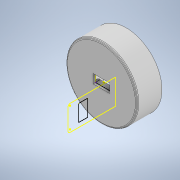
# Autodesk Inventor part: Base
Saved by Autodesk Inventor 2020 (Build 240168000, 168)
## iProperties
Created: 2020-02-27
Part Number: Base
Material: Generic
Document SubType Name: Modeling
Designer: othscs164
Density: 1 g/cm^3
Appearance: Default
Author: othscs164
Autodesk Inventor part; units mm, degrees
ref_plane "YZ Plane" through (0, 0, 0) normal (1, 0, 0) x (0, 1, 0)
ref_plane "XZ Plane" through (0, 0, 0) normal (0, 1, 0) x (-1, 0, 0)
ref_plane "XY Plane" through (0, 0, 0) normal (0, 0, 1) x (1, 0, 0)
sketch "Sketch1" plane through (0, 0, 0) normal (0, 0, 1) x (1, 0, 0)
  circle A0 centre (0, 0) radius 41.275
  circle A1 centre (0, 0) radius 47.625
  dimension "d0" = 82.55
  dimension "d1" = 6.35
  constraints: 2 centre point, 1 coincident
  measures "d0" diameter of A0
  measures "d1" radial gap between concentric circles of A0 A1
extrude "Extrusion1" add sketch "Sketch1" along normal blind 25.4
sketch "Sketch2" plane through (0, 0, 25.4) normal (0, 0, 1) x (1, 0, 0)
  circle A0 centre (0, 0) radius 47.625
  constraints: 1 centre point, 1 coincident
extrude "Extrusion2" add sketch "Sketch2" along normal blind 3.175
sketch "Sketch3" plane through (0, 0, 25.4) normal (0, 0, -1) x (-1, 0, 0)
  line L0 (11, 6) -> (-11, 6)
  line L1 (-11, 6) -> (-11, -6)
  line L2 (-11, -6) -> (11, -6)
  line L3 (11, -6) -> (11, 6)
  line L4 (11, 6) -> (-11, -6) construction
  line L5 (-11, 6) -> (11, -6) construction
  line L6 (-10.6662, 8.8412) -> (10.6662, 8.8412)
  line L7 (13.8412, 5.6662) -> (13.8412, -5.6662)
  line L8 (10.6662, -8.8412) -> (-10.6662, -8.8412)
  line L9 (-13.8412, -5.6662) -> (-13.8412, 5.6662)
  arc A0 (-10.6662, 8.8412) -> (-13.8412, 5.6662) centre (-10.6662, 5.6662) ccw
  arc A1 (-13.8412, -5.6662) -> (-10.6662, -8.8412) centre (-10.6662, -5.6662) ccw
  arc A2 (10.6662, -8.8412) -> (13.8412, -5.6662) centre (10.6662, -5.6662) ccw
  arc A3 (13.8412, 5.6662) -> (10.6662, 8.8412) centre (10.6662, 5.6662) ccw
  point P0 (0, 0)
  dimension "d6" = 22
  dimension "d7" = 12
  dimension "d8" = 3.175
  constraints: 20 end point, 8 point on circle, 8 tangent, 4 centre point, 4 parallel, 3 equal radius, 2 midpoint, 2 perpendicular, 1 horizontal, 3 other
  measures "d6" distance of L2.end L1.end
  measures "d7" distance of L1.end L0.end
  measures "d8" radius of A0
extrude "Extrusion3" add sketch "Sketch3" along normal blind 6.35
chamfer "Chamfer1" distance 1.5875 angle 45 8 edges at (0, 8.8412, 19.05) (12.9113, 7.9113, 19.05) (13.8412, 0, 19.05) (12.9113, -7.9113, 19.05) (0, -8.8412, 19.05) (-12.9113, -7.9113, 19.05) (-13.8412, 0, 19.05) (-12.9113, 7.9113, 19.05)
sketch "Sketch5" plane through (-13.8412, -5.6662, 25.4) normal (-1, 0, 0) x (0, 0, 1)
  line L0 (-0.1094, 0) -> (-8.0486, 0)
  line L1 (-8.0486, 0) -> (-8.0486, 11.3324)
  line L2 (-8.0486, 11.3324) -> (-0.1094, 11.3324)
  line L3 (-0.1094, 11.3324) -> (-0.1094, 0)
  point P0 (-25.4, 5.6662)
  constraints: 8 end point, 2 parallel, 1 horizontal, 1 perpendicular
extrude "Extrusion5" cut sketch "Sketch5" against normal blind 28.575
sketch "Sketch6" plane through (0, 0, 0) normal (0, 0, -1) x (-1, 0, 0)
  circle A0 centre (0, 0) radius 47.625 projected
  circle A1 centre (0, 0) radius 41.275 projected
extrude "Extrusion6" add sketch "Sketch6" along normal blind 4.5
chamfer "Chamfer2" distance 1.5875 angle 45 1 edges at (-47.625, 0, 28.575)
fillet "Fillet2" radius 1.5875 1 edges at (-46.0375, 0, 28.575)
fillet "Fillet3" radius 1.5875 1 edges at (-47.625, 0, 26.9875)
sketch "Sketch7" plane through (0, 0, 25.4) normal (0, 0, -1) x (-1, 0, 0)
  circle A0 centre (0, 0) radius 41.275 projected
  line L0 (-10.6662, 8.8412) -> (10.6662, 8.8412) projected
  arc A1 (13.8412, 5.6662) -> (10.6662, 8.8412) centre (10.6662, 5.6662) ccw projected
  line L1 (13.8412, 5.6662) -> (13.8412, -5.6662) projected
  arc A2 (10.6662, -8.8412) -> (13.8412, -5.6662) centre (10.6662, -5.6662) ccw projected
  line L2 (10.6662, -8.8412) -> (-10.6662, -8.8412) projected
  arc A3 (-13.8412, -5.6662) -> (-10.6662, -8.8412) centre (-10.6662, -5.6662) ccw projected
  line L3 (-13.8412, -5.6662) -> (-13.8412, 5.6662) projected
  arc A4 (-10.6662, 8.8412) -> (-13.8412, 5.6662) centre (-10.6662, 5.6662) ccw projected
  line L4 (10.6662, 7.2537) -> (10.6662, 8.8412) projected
  arc A5 (12.2537, 5.6662) -> (10.6662, 7.2537) centre (10.6662, 5.6662) ccw projected
  line L5 (13.8412, 5.6662) -> (12.2537, 5.6662) projected
  arc A6 (13.8412, 5.6662) -> (10.6662, 8.8412) centre (10.6662, 5.6662) ccw projected
  line L6 (-10.6662, 7.2537) -> (10.6662, 7.2537) projected
  line L7 (-12.2537, 5.6662) -> (-11, 5.6662) projected
  line L8 (-11, 5.6662) -> (-11, 6) projected
  line L9 (-11, 6) -> (11, 6) projected
  line L10 (11, 6) -> (11, 5.6662) projected
  line L11 (11, 5.6662) -> (12.2537, 5.6662) projected
  arc A7 (12.2537, 5.6662) -> (10.6662, 7.2537) centre (10.6662, 5.6662) ccw projected
  line L12 (-10.6662, 7.2537) -> (10.6662, 7.2537) projected
  arc A8 (-10.6662, 7.2537) -> (-12.2537, 5.6662) centre (-10.6662, 5.6662) ccw projected
  line L13 (-10.6662, 8.8412) -> (-10.6662, 7.2537) projected
  line L14 (-10.6662, 7.2537) -> (10.6662, 7.2537) projected
  line L15 (10.6662, 7.2537) -> (10.6662, 8.8412) projected
  line L16 (10.6662, 8.8412) -> (-10.6662, 8.8412) projected
  line L17 (-11, 6) -> (11, 6) projected
  line L18 (10.6662, 8.8412) -> (-10.6662, 8.8412) projected
  line L19 (11, 5.6662) -> (12.2537, 5.6662) projected
  line L20 (10.6662, 8.8412) -> (-10.6662, 8.8412)
  line L21 (-10.6662, -8.8412) -> (10.6662, -8.8412) projected
  line L22 (10.6662, -8.8412) -> (-10.6662, -8.8412)
  arc A9 (13.8412, 5.6662) -> (10.6662, 8.8412) centre (10.6662, 5.6662) ccw projected
  arc A10 (13.8412, 5.6662) -> (10.6662, 8.8412) centre (10.6662, 5.6662) ccw
  line L23 (10.6662, -8.8412) -> (10.6662, -7.2537) projected
  arc A11 (10.6662, -8.8412) -> (13.8412, -5.6662) centre (10.6662, -5.6662) ccw
  arc A12 (-13.8412, -5.6662) -> (-10.6662, -8.8412) centre (-10.6662, -5.6662) ccw
  arc A13 (-10.6662, 8.8412) -> (-13.8412, 5.6662) centre (-10.6662, 5.6662) ccw projected
  arc A14 (-10.6662, 8.8412) -> (-13.8412, 5.6662) centre (-10.6662, 5.6662) ccw
  line L24 (11, -6) -> (11, 6) projected
  line L25 (11, 5.6662) -> (11, 6)
  line L26 (11, 6) -> (-11, 6)
  line L27 (-11, 5.6662) -> (-11, -5.6662) projected
  line L28 (-11, 6) -> (-11, 5.6662)
  line L29 (-11, 5.6662) -> (-13.8412, 5.6662)
  line L30 (-11, -5.6662) -> (-13.8412, -5.6662) projected
  line L31 (-13.8412, -5.6662) -> (-11, -5.6662)
  line L32 (-11, -6) -> (-11, -5.6662) projected
  line L33 (-11, -5.6662) -> (-11, -6)
  line L34 (-11, -6) -> (11, -6)
  line L35 (11, -5.6662) -> (11, -6) projected
  line L36 (11, -6) -> (11, -5.6662)
  line L37 (13.8412, -5.6662) -> (11, -5.6662) projected
  line L38 (11, -5.6662) -> (13.8412, -5.6662)
  line L39 (10.6662, 7.2537) -> (10.6662, 8.8412) projected
  arc A15 (13.8412, 5.6662) -> (10.6662, 8.8412) centre (10.6662, 5.6662) ccw
  arc A16 (-10.6662, 8.8412) -> (-13.8412, 5.6662) centre (-10.6662, 5.6662) ccw
  line L40 (10.6662, 8.8412) -> (-10.6662, 8.8412)
  line L41 (11, 6) -> (-11, 6)
  line L42 (-11, 5.6662) -> (-11, 6)
  line L43 (-13.8412, 5.6662) -> (-12.2537, 5.6662) projected
  line L44 (-11, 5.6662) -> (-13.8412, 5.6662)
  line L45 (13.8412, 5.6662) -> (13.8412, -5.6662) projected
  line L46 (13.8412, 5.6662) -> (11, 5.6662)
  constraints: 32 end point, 13 point on circle, 6 centre point, 6 perpendicular, 4 collinear, 4 tangent, 2 concentric, 2 horizontal, 2 point on line, 2 vertical, 1 parallel
sketch "Sketch8" plane through (0, 0, 28.575) normal (0, 0, 1) x (1, 0, 0)
  line L0 (0, 0) -> (18.6341, 0)
  line L1 (18.6341, 0) -> (18.6341, -16.7894)
  line L2 (18.6341, -16.7894) -> (18.6341, 0)
  line L3 (18.6341, 0) -> (18.6341, 16.7894)
  line L4 (18.6341, 16.7894) -> (24.9841, 16.7894)
  line L5 (24.9841, 16.7894) -> (24.9841, -16.7894)
  line L6 (24.9841, -16.7894) -> (18.6341, -16.7894)
  dimension "d28" = 16.7894
  dimension "d29" = 6.35
  dimension "d30" = 33.5788
  constraints: 14 end point, 5 perpendicular, 1 horizontal, 1 point on line
  measures "d28" distance of L0.end L3.end
  measures "d29" distance of L3.end L4.end
  measures "d30" distance of L4.end L5.end
extrude "Extrusion7" add sketch "Sketch8" along normal blind 63.5
fillet "Fillet4" radius 3.175 3 edges at (24.9841, 0, 92.075) (21.8091, -16.7894, 92.075) (21.8091, 16.7894, 92.075)
sketch "Sketch10" plane through (0, 0, 25.4) normal (0, 0, -1) x (-1, 0, 0)
  line L0 (11, 6) -> (-11, 6) projected
  line L1 (-11, -6) -> (11, -6) projected
  line L2 (-11, 6) -> (11, 6)
  line L3 (11, 6) -> (11, -6)
  line L4 (11, -6) -> (-11, -6)
  line L5 (-11, -6) -> (-11, 6)
  point P0 (0, 0)
  constraints: 8 end point, 2 parallel, 1 horizontal, 1 perpendicular
extrude "Extrusion9" cut sketch "Sketch10" against normal up to surface (3.175 mm away)
sketch "Sketch11" plane through (18.6341, -16.7894, 28.575) normal (-1, 0, 0) x (0, 0, 1)
  line L0 (48.8213, 27.8052) -> (49.1551, 27.8061) projected
  line L1 (37.2166, 5.7727) -> (37.1859, 16.7726) projected
  line L2 (49.1551, 27.8061) -> (37.2166, 27.8061)
  line L3 (37.2166, 27.8061) -> (37.2166, 5.7727)
  line L4 (37.2166, 5.7727) -> (49.1551, 5.7727)
  line L5 (49.1551, 5.7727) -> (49.1551, 27.8061)
  point P0 (-28.575, 16.7894)
  constraints: 8 end point, 2 parallel, 1 horizontal, 1 perpendicular
extrude "Extrusion10" cut sketch "Sketch11" against normal up to surface (6.35 mm away)
sketch "Sketch12" plane through (18.6341, -16.7894, 28.575) normal (-1, 0, 0) x (0, 0, 1)
  line L0 (37.2166, 5.7727) -> (37.2166, 27.8061) projected
  line L1 (37.2166, 27.8061) -> (49.1551, 27.8061) projected
  line L2 (49.1551, 27.8061) -> (49.1551, 5.7727) projected
  line L3 (49.1551, 5.7727) -> (37.2166, 5.7727) projected
  arc A0 (63.5, 30.4038) -> (60.325, 33.5788) centre (60.325, 30.4038) ccw projected
  line L4 (0, 33.5788) -> (60.325, 33.5788) projected
  line L5 (0, 0) -> (0, 33.5788) projected
  line L6 (0, 0) -> (60.325, 0) projected
  arc A1 (60.325, 0) -> (63.5, 3.175) centre (60.325, 3.175) ccw projected
  line L7 (63.5, 30.4038) -> (63.5, 3.175) projected
  line L8 (37.2166, 27.8061) -> (37.2166, 5.7727) projected
  line L9 (49.1551, 27.8061) -> (37.2166, 27.8061)
  line L10 (37.2166, 27.8061) -> (37.2166, 5.7727)
  line L11 (37.2166, 5.7727) -> (49.1551, 5.7727)
  line L12 (49.1551, 5.7727) -> (49.1551, 27.8061)
  point P0 (-28.575, 16.7894)
  constraints: 8 end point, 2 parallel, 1 horizontal, 1 perpendicular
sketch "Sketch13" plane through (0, 0, 92.075) normal (0, 0, 1) x (1, 0, 0)
  circle A0 centre (0, 0) radius 41.275 projected
  line L0 (34.9461, 21.9635) -> (13.1232, 21.9635)
  line L1 (13.1232, 21.9635) -> (13.1232, -23.4108)
  line L2 (13.1232, -23.4108) -> (34.9461, -23.4108)
  line L3 (34.9461, -23.4108) -> (34.9461, 21.9635)
  point P0 (33.9936, -23.4108)
  point P1 (34.9461, -21.9635)
  constraints: 8 end point, 2 parallel, 1 horizontal, 1 perpendicular, 2 other
extrude "Extrusion11" cut sketch "Sketch13" against normal up to surface (63.5 mm away) contours L3 A0 L2 L1 L0
body "Solid1"
